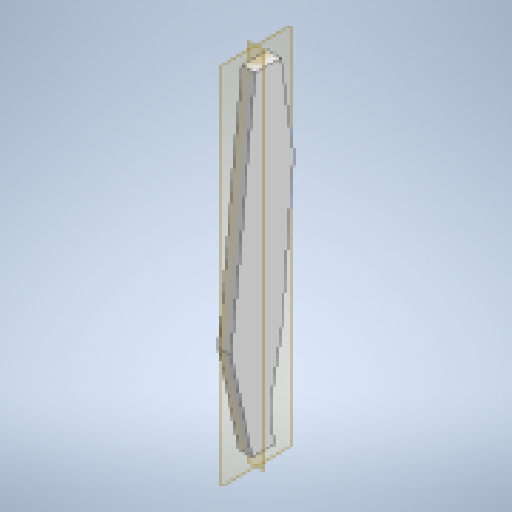
# Autodesk Inventor part: ForearmBoundingBOx
Saved by Autodesk Inventor 2023 (Build 270158000, 158)
## iProperties
Created: 2023-03-18
Part Number: ForearmBoundingBOx
Material: Generic
Document SubType Name: Modeling
Designer: Val
Density: 1 g/cm^3
Appearance: Default
Author: Val
Autodesk Inventor part; units mm, degrees
ref_plane "XZ Plane" through (0, 0, 0) normal (0, 1, 0) x (-1, 0, 0)
sketch "BoundingBox" plane through (0, 0, 0) normal (1, 0, 0) x (0, 1, 0)
  line L0 (-19.5, 16) -> (-19.5, -18)
  line L1 (-19.5, -18) -> (354.5938, -48.3648)
  line L2 (354.5938, -48.3648) -> (493.0939, -28.1898)
  line L3 (493.0939, -28.1898) -> (493.0939, 11.5)
  line L4 (493.0939, 11.5) -> (132.7202, 48.3)
  line L5 (132.7202, 48.3) -> (-19.5, 16)
  circle A0 centre (354.5938, -31.3648) radius 3.175 construction
  line L6 (354.5938, -48.3648) -> (354.5938, -31.3648) construction
  point P0 (0, 0)
  point P1 (0, 0)
  point P2 (480.5939, 0)
  point P3 (0, 0)
  point P4 (480.5939, 0)
  point P5 (60.5718, 4.3926)
  point P6 (60.5718, 4.3926)
  dimension "d0" = 19.5
  dimension "d1" = 101.98
  dimension "d2" = 18
  dimension "d3" = 16
  dimension "d4" = 12.5
  dimension "d5" = 11.5
  dimension "d6" = 48.3
  dimension "d7" = 39.6898
  dimension "d8" = 17
  dimension "d11" = 480.5939
  constraints: 14 end point, 3 coincident, 3 vertical, 1 centre point, 1 other
  measures "d0" distance from line of L0 point (0, 0)
  measures "d1" angle of L5 L0
  measures "d2" vertical distance of L0.end point (0, 0)
  measures "d3" vertical distance of L0.start point (0, 0)
  measures "d4" distance from line of L3 point (480.594, 0)
  measures "d5" vertical distance of L3.end point (480.594, 0)
  measures "d6" vertical distance of point (0, 0) L4.end
  measures "d7" distance of L2.end L3.end
  measures "d8" distance of L1.end L6.end
  measures "d11" distance of point (480.594, 0) point (0, 0)
extrude "BoundingBoxFeature" add sketch "BoundingBox" along normal mid plane 20.32
sketch "Sketch2" plane through (10.16, 0, 0) normal (1, 0, 0) x (0, 0, -1)
  line L0 (18, -19.5) -> (48.3648, 354.5938) projected
  line L1 (48.3648, 354.5938) -> (28.1898, 493.0939) projected
  line L2 (28.1898, 493.0939) -> (-11.5, 493.0939) projected
  line L3 (-11.5, 493.0939) -> (-48.3, 132.7202) projected
  line L4 (-48.3, 132.7202) -> (-16, -19.5) projected
  line L5 (-16, -19.5) -> (18, -19.5) projected
  arc A0 (-14.9278, 11.8349) -> (11.9767, 14.8142) centre (0, 0) ccw construction
  spline S0 degree 3 poles (12.7057, 41.3075) (12.6414, 56.2569) (13.3397, 71.2032) (14.7987, 86.0881) knots -4.923013 -4.923013 -4.923013 -4.923013 -0.435331 -0.435331 -0.435331 -0.435331 construction
  arc A1 (12.7313, 39.6054) -> (13.6561, 14.3145) centre (450.618, 42.9547) ccw construction
  line L6 (13.6561, 14.3145) -> (18, -19.5)
  line L7 (13.6561, 14.3145) -> (12.7057, 41.3075)
  line L8 (12.7057, 41.3075) -> (30.7136, 137.1318)
  line L9 (30.7136, 137.1318) -> (18, -19.5)
  point P0 (0, 0)
  constraints: 8 end point, 1 point on line
extrude "Extrusion2" cut sketch "Sketch2" along normal through all both and the other way through all contours L6 L7 L8 L0
body "Solid1"
